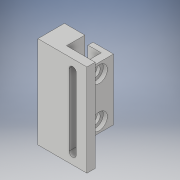
# Autodesk Inventor part: Schlitten_Part2
Saved by Autodesk Inventor 2019 (Build 230136000, 136)
## iProperties
Created: 2021-05-01
Part Number: Schlitten_Part2
Material: Generisch
Document SubType Name: Modeling
Designer: Bergi
Density: 1 g/cm^3
Appearance: Vorgabe
Author: Bergi
Autodesk Inventor part; units mm, degrees
ref_plane "YZ Plane" through (0, 0, 0) normal (1, 0, 0) x (0, 1, 0)
ref_plane "XZ Plane" through (0, 0, 0) normal (0, 1, 0) x (-1, 0, 0)
ref_plane "XY Plane" through (0, 0, 0) normal (0, 0, 1) x (1, 0, 0)
sketch "Skizze1" plane through (0, 0, 0) normal (0, 1, 0) x (-1, 0, 0)
  line L0 (-5, 7) -> (5, 7)
  line L1 (5, 7) -> (5, -7)
  line L2 (5, -7) -> (-5, -7)
  line L3 (-5, -7) -> (-5, 7)
  line L4 (-5, 7) -> (5, -7) construction
  line L5 (5, 7) -> (-5, -7) construction
  line L6 (5, 4.5) -> (-1.5, 4.5)
  line L7 (-1.5, 4.5) -> (-1.5, -4.5)
  line L8 (-1.5, -4.5) -> (5, -4.5)
  line L9 (5, -4.5) -> (5, 4.5)
  line L10 (5, 4.5) -> (-1.5, -4.5) construction
  line L11 (-1.5, 4.5) -> (5, -4.5) construction
  line L12 (7, 0) -> (-7, 0) projected
  point P0 (0, 0)
  point P1 (1.75, 0)
  point P2 (1.75, 0)
  dimension "d0" = 10
  dimension "d1" = 14
  dimension "d2" = 6.5
  dimension "d3" = 9
  constraints: 24 end point, 5 midpoint, 4 parallel, 2 horizontal, 2 perpendicular, 2 point on line
  measures "d0" distance of L1.end L2.end
  measures "d1" distance of L0.end L1.end
  measures "d2" distance of L8.end L7.end
  measures "d3" distance of L7.end L6.end
extrude "Extrusion1" add sketch "Skizze1" along normal blind 30 contours L0 L1 L6 L7 L12 L3 | L12 L7 L8 L1 L2 L3
sketch "Skizze2" plane through (5, 0, 7) normal (1, 0, 0) x (0, 0, -1)
  line L0 (7, -6) -> (7, 36) construction
  point P0 (7, 0)
  point P1 (7, 25)
  point P2 (7, 5)
  dimension "d6" = 20
  dimension "d7" = 5
  constraints: 2 point on line
  measures "d6" distance of point (7, 5) point (7, 25)
  measures "d7" distance of point (7, 0) point (7, 5)
hole "Bohrung1" at (5, 25, 0) at (5, 5, 0) direction (-1, 0, 0) diameter 5 end through all counterbore diameter 8 counterbore depth 2
sketch "Skizze3" plane through (0, 30, 0) normal (0, 1, 0) x (1, 0, 0)
  line L0 (-5, 4.5) -> (1.5, 4.5) projected
  line L1 (1.5, 4.5) -> (1.5, -4.5) projected
  line L2 (1.5, -4.5) -> (-5, -4.5) projected
  line L3 (-5, -4.5) -> (-5, -7) projected
  line L4 (-5, -7) -> (5, -7) projected
  line L5 (5, -7) -> (5, 7) projected
  line L6 (5, 7) -> (-5, 7) projected
  line L7 (-5, 7) -> (-5, 4.5) projected
  line L8 (5, 7) -> (-5, 7) projected
  line L9 (-5, -7) -> (-5, -20)
  line L10 (-5, -20) -> (19, -20)
  line L11 (19, -20) -> (19, -16)
  line L12 (19, -16) -> (5, -16)
  line L13 (5, -7) -> (5, 7) projected
  line L14 (5, -16) -> (5, -7)
  point P0 (0, 0)
  dimension "d16" = 20
  dimension "d17" = 14
  dimension "d18" = 4
  constraints: 10 end point, 3 perpendicular, 1 collinear, 1 point on line, 1 vertical
  measures "d16" distance from line of point (0, 0) L10
  measures "d17" distance between parallel lines of L5 L11
  measures "d18" distance of L10.end L11.end
extrude "Extrusion2" add sketch "Skizze3" against normal blind 30 and the other way blind 15 contours L14 L12 L11 L10 L9 L4
sketch "Skizze4" plane through (19, 0, 16) normal (0, 0, -1) x (-1, 0, 0)
  line L0 (0, 0) -> (0, 45) projected
  line L1 (14, 0) -> (0, 0) projected
  line L2 (14, 0) -> (14, 45) projected
  line L3 (0, 45) -> (14, 45) projected
  line L4 (24, 45) -> (0, 45) projected
  line L5 (7, 45) -> (7, 0) construction
  line L6 (14, 0) -> (0, 0) projected
  line L7 (7, 40) -> (7, 5) construction
  line L8 (5.25, 40) -> (5.25, 5)
  line L9 (8.75, 5) -> (8.75, 40)
  arc A0 (8.75, 40) -> (5.25, 40) centre (7, 40) ccw
  arc A1 (5.25, 5) -> (8.75, 5) centre (7, 5) ccw
  point P0 (19, 0)
  point P1 (7, 22.5)
  dimension "d23" = 3.5
  dimension "d24" = 5
  dimension "d25" = 5
  constraints: 10 end point, 4 point on circle, 4 tangent, 3 point on line, 2 centre point, 2 midpoint, 1 parallel
  measures "d23" diameter of A1
  measures "d24" distance from line of L3 L8.start
  measures "d25" distance from line of L1 L8.end
extrude "Extrusion3" cut sketch "Skizze4" against normal blind 30 contours A0 L9 A1 L8
